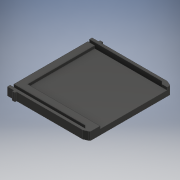
# Autodesk Inventor part: TA10
Saved by Autodesk Inventor 2017 (Build 210142000, 142)
## iProperties
Created: 2019-04-23
Part Number: TA10
Material: ABS Plastic
Document SubType Name: Modeling
Designer: Dell
Density: 1.06 g/cm^3
Appearance: Smooth - Black
Author: Dell
Autodesk Inventor part; units mm, degrees
ref_plane "YZ Plane" through (0, 0, 0) normal (1, 0, 0) x (0, 1, 0)
ref_plane "XZ Plane" through (0, 0, 0) normal (0, 1, 0) x (-1, 0, 0)
ref_plane "XY Plane" through (0, 0, 0) normal (0, 0, 1) x (1, 0, 0)
sketch "Sketch1" plane through (0, 0, 0) normal (0, 0, 1) x (1, 0, 0)
  line L0 (0, 0) -> (30, 0)
  line L1 (30, 0) -> (30, 30)
  line L2 (30, 30) -> (0, 30)
  line L3 (0, 30) -> (0, 0)
  dimension "d0" = 30
  dimension "d1" = 30
  constraints: 8 end point, 2 parallel, 1 horizontal, 1 perpendicular
  measures "d0" distance of L1.end L0.end
  measures "d1" distance of L1.end L2.end
extrude "Extrusion1" add sketch "Sketch1" along normal blind 3
sketch "Sketch2" plane through (0, 0, 3) normal (0, 0, 1) x (1, 0, 0)
  line L0 (30, 3.6) -> (2.6, 3.6)
  line L1 (2.6, 3.6) -> (2.6, 29)
  line L2 (2.6, 29) -> (30, 29)
  line L3 (30, 29) -> (30, 3.6)
  line L4 (0, 0) -> (30, 0) projected
  line L5 (30, 0) -> (30, 30) projected
  dimension "d4" = 27.4
  dimension "d5" = 25.4
  dimension "d36" = 3.6
  constraints: 8 end point, 2 parallel, 1 horizontal, 1 perpendicular, 1 point on line
  measures "d4" distance of L1.end L2.end
  measures "d5" distance of L0.end L1.end
  measures "d36" distance between parallel lines of L4 L0
extrude "Extrusion2" cut sketch "Sketch2" against normal blind 1
sketch "Sketch3" plane through (0, 0, 3) normal (0, 0, 1) x (1, 0, 0)
  line L0 (30, 30) -> (0, 30) projected
  line L1 (0, 30) -> (0, 0) projected
  line L2 (28, 30) -> (0, 30)
  line L3 (0, 30) -> (0, 29)
  line L4 (0, 29) -> (28, 29)
  line L5 (28, 29) -> (28, 30)
  line L6 (30, 29) -> (30, 30) projected
  line L7 (0, 0) -> (30, 0) projected
  line L8 (28, 0) -> (0, 0)
  line L9 (0, 0) -> (0, 1)
  line L10 (0, 1) -> (28, 1)
  line L11 (28, 1) -> (28, 0)
  line L12 (30, 0) -> (30, 3.6) projected
  dimension "d8" = 1
  dimension "d9" = 2
  dimension "d10" = 1
  dimension "d11" = 2
  constraints: 16 end point, 4 parallel, 4 point on line, 2 horizontal, 2 perpendicular
  measures "d8" distance of L4.end L2.start
  measures "d9" distance between parallel lines of L6 L5
  measures "d10" distance of L10.end L8.start
  measures "d11" distance between parallel lines of L12 L11
extrude "Extrusion3" cut sketch "Sketch3" against normal through all
sketch "Sketch4" plane through (0, 0, 3) normal (0, 0, 1) x (1, 0, 0)
  line L0 (30, 29) -> (30, 30) projected
  line L1 (30, 30) -> (-0.4, 30)
  line L2 (-0.4, 30) -> (-0.4, 31)
  line L3 (-0.4, 31) -> (30, 31)
  line L4 (30, 31) -> (30, 30)
  line L5 (30, 0) -> (-0.4, 0)
  line L6 (-0.4, 0) -> (-0.4, -1)
  line L7 (-0.4, -1) -> (30, -1)
  line L8 (30, -1) -> (30, 0)
  line L9 (2, 31) -> (3, 31)
  line L10 (3, 31) -> (3, 31.6)
  line L11 (3, 31.6) -> (2, 31.6)
  line L12 (2, 31.6) -> (2, 31)
  line L13 (2, -1) -> (3, -1)
  line L14 (3, -1) -> (3, -1.6)
  line L15 (3, -1.6) -> (2, -1.6)
  line L16 (2, -1.6) -> (2, -1)
  line L17 (0, 29) -> (0, 1) projected
  point P0 (0, 0)
  dimension "d14" = 30.4
  dimension "d15" = 1
  dimension "d17" = 1
  dimension "d20" = 1
  dimension "d21" = 0.6
  dimension "d26" = 1
  dimension "d27" = 0.6
  dimension "d35" = 2
  constraints: 32 end point, 8 parallel, 4 horizontal, 4 perpendicular, 3 point on line, 2 vertical alignment, 1 coincident
  measures "d14" distance of L2.end L3.end
  measures "d15" distance of L1.end L2.end
  measures "d17" distance of L6.end L5.end
  measures "d20" distance of L11.end L10.end
  measures "d21" distance of L10.end L9.end
  measures "d26" distance of L14.end L15.end
  measures "d27" distance of L13.end L14.end
  measures "d35" distance between parallel lines of L12 L17
extrude "Extrusion4" add sketch "Sketch4" against normal blind 3
chamfer "Chamfer1" distance 1 angle 45 4 edges at (30, 31, 1.5) (30, -1, 1.5) (28, 1, 1.5) (28, 30, 1.5)
chamfer "Chamfer2" distance 1 angle 45 2 edges at (29.0001, 31, 1.5) (29.0001, -1, 1.5)
body "Solid1"
